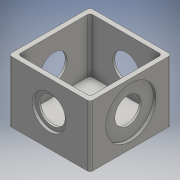
# Autodesk Inventor part: sampleChamber_singlePiece_filipeSample_V2
Saved by Autodesk Inventor 2016 (Build 200138000, 138)
## iProperties
Created: 2016-07-14
Part Number: sampleChamber_singlePiece_filipeSample_V2
Material: Generic
Document SubType Name: Modeling
Designer: sims01
Density: 1 g/cm^3
Appearance: Default
Author: sims01
Autodesk Inventor part; units mm, degrees
ref_plane "YZ Plane" through (0, 0, 0) normal (1, 0, 0) x (0, 1, 0)
ref_plane "XZ Plane" through (0, 0, 0) normal (0, 1, 0) x (-1, 0, 0)
ref_plane "XY Plane" through (0, 0, 0) normal (0, 0, 1) x (1, 0, 0)
sketch "Sketch1" plane through (0, 0, 0) normal (0, 0, 1) x (1, 0, 0)
  line L0 (-28, 30) -> (28, 30)
  line L1 (30, 28) -> (30, -28)
  line L2 (28, -30) -> (-28, -30)
  line L3 (-30, -28) -> (-30, 28)
  arc A0 (-28, 30) -> (-30, 28) centre (-28, 28) ccw
  arc A1 (-30, -28) -> (-28, -30) centre (-28, -28) ccw
  arc A2 (28, -30) -> (30, -28) centre (28, -28) ccw
  arc A3 (30, 28) -> (28, 30) centre (28, 28) ccw
  point P0 (0, 0)
  point P1 (-30, 30)
  point P2 (30, -30)
  point P3 (30, 30)
  dimension "d0" = 60
  dimension "d1" = 60
  dimension "d2" = 30
  dimension "d3" = 30
  dimension "d4" = 2
  constraints: 8 end point, 8 point on circle, 8 tangent, 6 point on line, 4 centre point, 3 equal radius, 2 parallel, 1 horizontal, 1 perpendicular
  measures "d0" distance of point (-30, 30) point (30, 30)
  measures "d1" distance of point (30, 30) point (30, -30)
  measures "d2" distance from line of point (0, 0) L1
  measures "d3" distance from line of point (0, 0) L0
  measures "d4" radius of A0
extrude "Extrusion1" add sketch "Sketch1" along normal blind 45
sketch "Sketch2" plane through (0, 0, 45) normal (0, 0, 1) x (1, 0, 0)
  line L0 (-24.5, 26.5) -> (24.5, 26.5)
  line L1 (26.5, 24.5) -> (26.5, -24.5)
  line L2 (24.5, -26.5) -> (-24.5, -26.5)
  line L3 (-26.5, -24.5) -> (-26.5, 24.5)
  arc A0 (-24.5, 26.5) -> (-26.5, 24.5) centre (-24.5, 24.5) ccw
  arc A1 (-26.5, -24.5) -> (-24.5, -26.5) centre (-24.5, -24.5) ccw
  arc A2 (24.5, -26.5) -> (26.5, -24.5) centre (24.5, -24.5) ccw
  arc A3 (26.5, 24.5) -> (24.5, 26.5) centre (24.5, 24.5) ccw
  point P0 (0, 0)
  point P1 (-26.5, 26.5)
  point P2 (26.5, -26.5)
  point P3 (26.5, 26.5)
  dimension "d7" = 53
  dimension "d8" = 53
  dimension "d9" = 26.5
  dimension "d10" = 26.5
  dimension "d11" = 2
  constraints: 8 end point, 8 point on circle, 8 tangent, 6 point on line, 4 centre point, 3 equal radius, 2 parallel, 1 horizontal, 1 perpendicular
  measures "d7" distance of point (-26.5, 26.5) point (26.5, 26.5)
  measures "d8" distance of point (26.5, 26.5) point (26.5, -26.5)
  measures "d9" distance from line of point (0, 0) L0
  measures "d10" distance from line of point (0, 0) L1
  measures "d11" radius of A0
extrude "Extrusion2" cut sketch "Sketch2" against normal blind 40
sketch "Sketch3" plane through (30, -28, 0) normal (1, 0, 0) x (0, 0, -1)
  circle A0 centre (-23.5, 28) radius 18.5
  line L0 (0, 0) -> (0, 56) projected
  point P0 (0, 28)
  point P1 (0, 28)
  dimension "d14" = 37
  dimension "d15" = 23.5
  constraints: 1 centre point, 1 horizontal alignment, 1 midpoint
  measures "d14" diameter of A0
  measures "d15" distance from line of L0 A0.centre
extrude "Extrusion3" cut sketch "Sketch3" against normal blind 2
mirror "Mirror1" about plane through (0, 0, 0) normal (1, 0, 0) of "Extrusion3"
sketch "Sketch4" plane through (-28, 30, 0) normal (0, 1, 0) x (1, 0, 0)
  circle A0 centre (28, -23.5) radius 12.5
  point P0 (28, 0)
  dimension "d18" = 25
  dimension "d19" = 23.5
  constraints: 1 centre point
  measures "d18" diameter of A0
  measures "d19" distance of point (28, 0) A0.centre
extrude "Extrusion4" cut sketch "Sketch4" against normal blind 2
mirror "Mirror2" about plane through (0, 0, 0) normal (0, 1, 0) of "Extrusion4"
sketch "Sketch5" plane through (-28, 0, 23.5) normal (-1, 0, 0) x (0, 0, 1)
  circle A0 centre (0, 0) radius 9.75
  circle A1 centre (0, 0) radius 18.5 projected
  point P0 (-23.5, 0)
  dimension "d22" = 19.5
  constraints: 1 centre point, 1 concentric
  measures "d22" diameter of A0
extrude "Extrusion5" cut sketch "Sketch5" against normal blind 2 contours A0
pattern_circular "Circular Pattern1" count 4 over 360 about axis through (0, 0, -10) along (0, 0, 1) of "Extrusion5"
equation "\"d2\" = 0.5 * d0"
equation "\"d3\" = 0.5 * d1"
equation "\"d9\" = 0.5 * d8"
equation "\"d10\" = 0.5 * d7"
body "Solid1"
